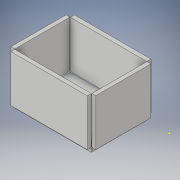
# Autodesk Inventor part: frame
Saved by Autodesk Inventor 2019 (Build 230136000, 136)
## iProperties
Created: 2020-02-19
Part Number: frame
Material: Generic
Document SubType Name: Sheet Metal
Designer: unusualgamer
Density: 1 g/cm^3
Sheet Metal Rule: Default_mm
Appearance: Default
Author: unusualgamer
Autodesk Inventor part; units mm, degrees
ref_plane "YZ Plane" through (0, 0, 0) normal (1, 0, 0) x (0, 1, 0)
ref_plane "XZ Plane" through (0, 0, 0) normal (0, 1, 0) x (-1, 0, 0)
ref_plane "XY Plane" through (0, 0, 0) normal (0, 0, 1) x (1, 0, 0)
sketch "Sketch1" plane through (0, 0, 0) normal (0, 1, 0) x (-1, 0, 0)
  line L0 (243.2018, 140.1406) -> (43.2018, 140.1406)
  line L1 (43.2018, 140.1406) -> (43.2018, -9.8594)
  line L2 (43.2018, -9.8594) -> (243.2018, -9.8594)
  line L3 (243.2018, -9.8594) -> (243.2018, 140.1406)
  point P0 (0, 0)
  dimension "d0" = 200
  dimension "d1" = 150
  constraints: 8 end point, 2 parallel, 1 horizontal, 1 perpendicular
  measures "d0" distance of L2.end L1.end
  measures "d1" distance of L1.end L0.end
extrude "Extrusion1" add sketch "Sketch1" along normal blind 120
sketch "Sketch2" plane through (0, 120, 0) normal (0, 1, 0) x (1, 0, 0)
  line L0 (-233.9237, -130.8252) -> (-52.3036, -130.8252)
  line L1 (-52.3036, -130.8252) -> (-52.3036, 0)
  line L2 (-52.3036, 0) -> (-233.9237, 0)
  line L3 (-233.9237, 0) -> (-233.9237, -130.8252)
  point P0 (0, 0)
  constraints: 8 end point, 2 parallel, 1 horizontal, 1 perpendicular
extrude "Extrusion2" cut sketch "Sketch2" against normal blind 110
sketch "Sketch3" plane through (-243.2018, 0, 140.1406) normal (0, 0, 1) x (1, 0, 0)
  line L0 (0, 0) -> (0, 120) projected
  line L1 (0, 0) -> (200, 0) projected
  line L2 (0, 120) -> (9.9841, 120)
  line L3 (9.9841, 120) -> (9.9841, 0)
  line L4 (9.9841, 0) -> (0, 0)
  line L5 (0, 0) -> (0, 120)
  point P0 (243.2018, 0)
  constraints: 8 end point, 2 parallel, 1 horizontal, 1 perpendicular, 1 point on line
extrude "Extrusion3" cut sketch "Sketch3" against normal blind 10
sketch "Sketch4" plane through (-43.2018, 0, 140.1406) normal (0, 0, 1) x (1, 0, 0)
  line L0 (0, 120) -> (-200, 120) projected
  line L1 (0, 0) -> (-200, 0) projected
  line L2 (0, 120) -> (-9.6366, 120)
  line L3 (-9.6366, 120) -> (-9.6366, 0)
  line L4 (-9.6366, 0) -> (0, 0)
  line L5 (0, 0) -> (0, 120)
  point P0 (43.2018, 0)
  constraints: 8 end point, 2 parallel, 1 horizontal, 1 perpendicular, 1 point on line
extrude "Extrusion4" cut sketch "Sketch4" against normal blind 10
sketch "Sketch5" plane through (-43.2018, 0, -9.8594) normal (0, 0, -1) x (-1, 0, 0)
  line L0 (0, 120) -> (200, 120) projected
  line L1 (190.0159, 0) -> (9.6366, 0) projected
  line L2 (0, 120) -> (9.6366, 120)
  line L3 (9.6366, 120) -> (9.6366, 0)
  line L4 (9.6366, 0) -> (0, 0)
  line L5 (0, 0) -> (0, 120)
  point P0 (-43.2018, 0)
  constraints: 8 end point, 2 parallel, 1 horizontal, 1 perpendicular
extrude "Extrusion5" cut sketch "Sketch5" against normal blind 10
sketch "Sketch6" plane through (-243.2018, 0, -9.8594) normal (0, 0, -1) x (-1, 0, 0)
  line L0 (0, 0) -> (0, 120) projected
  line L1 (-190.3634, 0) -> (0, 0) projected
  line L2 (0, 120) -> (-9.9841, 120)
  line L3 (-9.9841, 120) -> (-9.9841, 0)
  line L4 (-9.9841, 0) -> (0, 0)
  line L5 (0, 0) -> (0, 120)
  point P0 (-243.2018, 0)
  constraints: 8 end point, 2 parallel, 1 horizontal, 1 perpendicular, 1 point on line
extrude "Extrusion6" cut sketch "Sketch6" against normal blind 10
sketch "Sketch7" plane through (0, 0, 0) normal (0, -1, 0) x (1, 0, 0)
  point P0 (0, 0)
sketch "Sketch8" plane through (0, 0, 0) normal (0, -1, 0) x (1, 0, 0)
  line L0 (-233.2177, 130.1406) -> (-243.2018, 130.1406) projected
  line L1 (-243.2018, 0.1406) -> (-243.2018, 130.1406) projected
  line L2 (-233.2177, 130.1406) -> (-243.2018, 130.1406)
  line L3 (-243.2018, 130.1406) -> (-243.2018, 0.1406)
  line L4 (-243.2018, 0.1406) -> (-233.2177, 0.1406)
  line L5 (-233.2177, 0.1406) -> (-233.2177, 130.1406)
  point P0 (0, 0)
  constraints: 8 end point, 2 parallel, 1 horizontal, 1 perpendicular
extrude "Extrusion7" cut sketch "Sketch8" against normal blind 10
sketch "Sketch9" plane through (0, 0, 0) normal (0, -1, 0) x (1, 0, 0)
  line L0 (-43.2018, 130.1406) -> (-43.2018, 0.1406) projected
  line L1 (-233.2177, 0) -> (-52.8384, 0) projected
  line L2 (-43.2018, 130.1406) -> (-52.8384, 130.1406)
  line L3 (-52.8384, 130.1406) -> (-52.8384, 0)
  line L4 (-52.8384, 0) -> (-43.2018, 0)
  line L5 (-43.2018, 0) -> (-43.2018, 130.1406)
  point P0 (0, 0)
  constraints: 8 end point, 2 parallel, 1 horizontal, 1 perpendicular
extrude "Extrusion8" cut sketch "Sketch9" against normal blind 10
sketch "Sketch10" plane through (0, 0, 0) normal (0, -1, 0) x (1, 0, 0)
  line L0 (-233.2177, 0) -> (-52.8384, 0) projected
  line L1 (-233.2177, 140.1406) -> (-233.2177, -9.8594) projected
  line L2 (-52.8384, 0) -> (-233.2177, 0)
  line L3 (-233.2177, 0) -> (-233.2177, -9.8594)
  line L4 (-233.2177, -9.8594) -> (-52.8384, -9.8594)
  line L5 (-52.8384, -9.8594) -> (-52.8384, 0)
  point P0 (0, 0)
  constraints: 8 end point, 2 parallel, 1 horizontal, 1 perpendicular
extrude "Extrusion9" cut sketch "Sketch10" against normal blind 10
sketch "Sketch11" plane through (0, 0, 0) normal (0, -1, 0) x (1, 0, 0)
  line L0 (-52.8384, 140.1406) -> (-52.8384, 130.8252) projected
  line L1 (-52.8384, 130.8252) -> (-233.2177, 130.8252) projected
  line L2 (-52.8384, 140.1406) -> (-233.2177, 140.1406)
  line L3 (-233.2177, 140.1406) -> (-233.2177, 130.8252)
  line L4 (-233.2177, 130.8252) -> (-52.8384, 130.8252)
  line L5 (-52.8384, 130.8252) -> (-52.8384, 140.1406)
  point P0 (0, 0)
  constraints: 8 end point, 2 parallel, 1 horizontal, 1 perpendicular
extrude "Extrusion10" cut sketch "Sketch11" against normal blind 10
sketch "Sketch12" plane through (-52.8384, 0, 0) normal (0, 0, -1) x (-1, 0, 0)
  line L0 (0, 10) -> (0, 0) projected
  line L1 (180.3793, 10) -> (180.3793, 0) projected
  line L2 (0, 10) -> (180.3793, 10)
  line L3 (180.3793, 10) -> (180.3793, 8.0332)
  line L4 (180.3793, 8.0332) -> (0, 8.0332)
  line L5 (0, 8.0332) -> (0, 10)
  point P0 (-52.8384, 0)
  constraints: 8 end point, 2 parallel, 1 horizontal, 1 perpendicular, 1 point on line
extrude "Extrusion11" cut sketch "Sketch12" against normal through all
equation "\"BendRadius\" = Thickness"
equation "\"BendReliefWidth\" = Thickness"
equation "\"BendReliefDepth\" = 0.5 * Thickness"
equation "\"CornerReliefSize\" = 4 * Thickness"
equation "\"MinimumRemnant\" = 2 * Thickness"
equation "\"TransitionRadius\" = BendRadius"
equation "\"JacobiRadiusSize\" = BendRadius"
equation "\"GapSize\" = Thickness"
equation "\"Thickness\" = 0.5"
body "Solid1"
